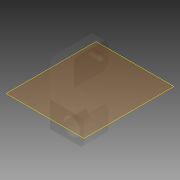
# Autodesk Inventor part: D-058
Saved by Autodesk Inventor 2015 (Build 190159000, 159)
## iProperties
Company: MARCHA TECHNOLOGY
Created: 2013-09-29
Part Number: D-058
Document SubType Name: Modeling
Designer: O.Martin
Density: 1.06 g/cm^3
Project: WITBOXprinter_K01
Description: SOPORTE TUBO TEFLON
Stock Number: 28655
Material: ABS Plastic
Mass: 9.94302 g
Surface Area: 41.9468 cm^2
Volume: 9.38021 cm^3
Appearance: Clear - Light
Author: O.Martin
Autodesk Inventor part; units mm, degrees
ref_plane "YZ Plane" through (0, 0, 0) normal (1, 0, 0) x (0, 1, 0)
ref_plane "XZ Plane" through (0, 0, 0) normal (0, 1, 0) x (-1, 0, 0)
sketch "Boceto1" plane through (0, 0, 0) normal (0, 0, 1) x (1, 0, 0)
  line L0 (7.5, 14) -> (-12.5, 14)
  line L1 (-26.5, 28) -> (-26.5, 48)
  line L2 (-26.5, 48) -> (-34, 48)
  line L3 (7.5, 0) -> (7.5, 14)
  line L4 (-1.9289, 0) -> (-1.9289, 16) construction
  arc A0 (-1.9289, 16) -> (-26.9289, 41) centre (-26.9289, 16) ccw construction
  line L5 (-26.9289, 41) -> (-54.881, 41) construction
  line L6 (2.0711, 0) -> (2.0711, 16) construction
  arc A1 (2.0711, 16) -> (-26.9289, 45) centre (-26.9289, 16) ccw construction
  line L7 (-26.9289, 45) -> (-54.881, 45) construction
  line L8 (-1.9289, 0) -> (2.0711, 0) construction
  line L9 (0.0711, 0) -> (0.0711, -17.3893) construction
  line L10 (-26.5, 28) -> (-12.5, 14)
  line L11 (7.5, 0) -> (-12.6421, 0)
  line L12 (-12.6421, 0) -> (-34, 21.3579)
  line L13 (-34, 48) -> (-34, 21.3579)
  point P0 (0, 0)
  dimension "d0" = 14
  dimension "d1" = 4
  dimension "d3" = 25
  dimension "d5" = 7.5
  dimension "d6" = 48
  dimension "d7" = 10
  dimension "d8" = 45
  dimension "d18" = 7.5
  dimension "d19" = 20
  dimension "d37" = 3
  constraints: 28 end point, 6 perpendicular, 5 parallel, 4 point on circle, 2 centre point, 2 point on line, 2 tangent, 1 horizontal, 1 midpoint, 2 other
  measures "d0" distance of L3.start L0.start
  measures "d1" distance between parallel lines of L5 L7
  measures "d3" radius of A0
  measures "d5" distance of L1.end L2.end
  measures "d6" distance between parallel lines of L11 L2
  measures "d7" distance between parallel lines of L12 L10
  measures "d8" angle of L12 L11
  measures "d18" distance from line of L3 point (0, 0)
  measures "d19" distance of L0.start L0.end
  measures "d37" distance between parallel lines of L2 L7
extrude "Extrusión1" add sketch "Boceto1" along normal mid plane 15
sketch "Boceto2" plane through (-12.6421, 0, 7.5) normal (0, -1, 0) x (1, 0, 0)
  line L0 (20.1421, -15) -> (20.1421, 0) projected
  circle A0 centre (12.6421, -7.5) radius 5
  point P0 (20.1421, -7.5)
  dimension "d11" = 10
  dimension "d12" = 7.5
  constraints: 1 centre point, 1 horizontal alignment, 1 midpoint
  measures "d11" diameter of A0
  measures "d12" distance from line of L0 A0.centre
extrude "Extrusión2" cut sketch "Boceto2" against normal through all
fillet "Empalme1" radius 5 2 edges at (-26.5, 28, 0) (-12.5, 14, 0)
fillet "Empalme1" radius 10 1 edges at (-34, 21.3579, 0)
sketch "Boceto4" plane through (-34, 25.5, -7.5) normal (-1, 0, 0) x (0, 0, 1)
  line L0 (15, 0) -> (15, 22.5) projected
  line L1 (9.5, 16.5) -> (9.5, 18)
  arc A0 (9.5, 18) -> (5.5, 18) centre (7.5, 18) ccw
  line L2 (5.5, 18) -> (5.5, 14.5)
  arc A1 (5.5, 14.5) -> (7.5, 12.5) centre (7.5, 14.5) ccw
  line L3 (7.5, 12.5) -> (15, 12.5)
  line L4 (0, 22.5) -> (15, 22.5) projected
  line L5 (0, 22.5) -> (0, 0) projected
  line L6 (9.5, 16.5) -> (15, 16.5)
  circle A2 centre (7.5, 18) radius 2
  point P0 (7.5, 22.5)
  dimension "d27" = 4
  dimension "d34" = 2.5
  dimension "d35" = 4
  dimension "d36" = 1.5
  constraints: 8 end point, 4 point on circle, 4 tangent, 3 centre point, 2 equal radius, 2 parallel, 2 perpendicular, 2 point on line, 1 coincident, 1 midpoint, 1 vertical alignment
  measures "d27" distance between parallel lines of L1 L2
  measures "d34" distance edge to line of A0 L4
  measures "d35" distance between parallel lines of L3 L6
  measures "d36" distance from line of A0.centre L6
extrude "Extrusión4" cut sketch "Boceto4" against normal blind 15 contours A2 A0
chamfer "Chaflán1" distance 2 angle 45 4 edges at (-30.25, 48, 7.5) (-30.25, 48, -7.5) (7.5, 7, 7.5) (7.5, 7, -7.5)
equation "\"d35\" = d27"
body "Solid1"
